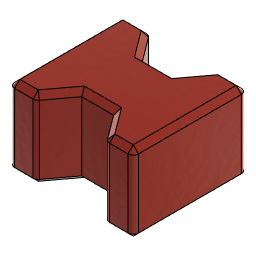
47 & 43mm Inner Frame Spacer Jig v6 (Autodesk Fusion 360 design; units mm, degrees)
Autodesk Fusion 360 part; units mm, degrees
sketch "Sketch1" plane through (0, 0, 0) normal (0, 1, 0) x (1, 0, 0)
  line L0 (47, 0) -> (47, -43)
  line L1 (0, -43) -> (0, 0)
  line L2 (10, -43) -> (17.4506, -33)
  line L3 (17.4506, -33) -> (29.5494, -33)
  line L4 (29.5494, -33) -> (37, -43)
  line L5 (0, -21.5) -> (47, -21.5) construction
  line L6 (47, -43) -> (37, -43)
  line L7 (10, -43) -> (0, -43)
  line L8 (10, 0) -> (17.4506, -10)
  line L9 (17.4506, -10) -> (29.5494, -10)
  line L10 (29.5494, -10) -> (37, 0)
  line L11 (0, 0) -> (10, 0)
  line L12 (37, 0) -> (47, 0)
  dimension "d1" = 47
  dimension "d2" = 43
  dimension "d6" = 23
  dimension "d10" = 10
  constraint horizontal L11
  constraint vertical L0
  constraint horizontal L6
  constraint vertical L1
  constraint coincident L1.end L11.start
  constraint coincident L2.start L6
  constraint perpendicular L1 L3
  constraint midpoint L1 L5.start
  constraint midpoint L0 L5.end
  constraint collinear L6 L7
  constraint equal L6 L7
  constraint symmetric L2.start L5 L8.start
  constraint symmetric L2.end L5 L8.end
  constraint symmetric L3.end L5 L9.end
  constraint symmetric L4.end L5 L10.end
  constraint equal L2 L4
  constraint collinear L11 L12
  measures "d1" distance of L1.end L0.start
  measures "d2" distance of L6 L11
  measures "d6" distance of L3 L9
  measures "d10" distance of L1 L2.start
extrude "Extrude1" add sketch "Sketch1" along normal blind 30
fillet "Fillet1" radius 2 8 edges at (0, 15, 43) (0, 15, 0) (47, 15, 0) (47, 15, 43) (10, 15, 43) (37, 15, 43) (10, 15, 0) (37, 15, 0)
chamfer "Chamfer2" distance 2 angle 45 2 faces at (5.8169, 0, 17.6667) (5.8169, 30, 17.6667)
move_body "Move1" bodies 1 to x (1, 0, 0) y (0, 0, 1) z (0, -1, 0) at (0, 21.5, 21.5)
equation "d2 = 47 mm - 4 mm"
